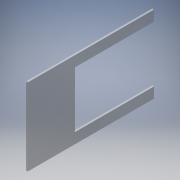
# Autodesk Inventor part: Inner side wall
Saved by Autodesk Inventor 2017 (Build 210142000, 142)
## iProperties
Created: 2017-09-30
Part Number: Inner side wall
Material: Glass
Document SubType Name: Modeling
Designer: Kenneth
Density: 2.18 g/cm^3
Appearance: Clear
Author: Kenneth
Autodesk Inventor part; units mm, degrees
ref_plane "YZ Plane" through (0, 0, 0) normal (1, 0, 0) x (0, 1, 0)
ref_plane "XZ Plane" through (0, 0, 0) normal (0, 1, 0) x (-1, 0, 0)
ref_plane "XY Plane" through (0, 0, 0) normal (0, 0, 1) x (1, 0, 0)
sketch "Sketch1" plane through (0, 0, 0) normal (1, 0, 0) x (0, 1, 0)
  line L0 (0, 0) -> (0, -457.2)
  line L1 (279.4, -457.2) -> (279.4, 0)
  line L2 (279.4, 0) -> (0, 0)
  line L3 (279.4, -457.2) -> (241.3, -457.2)
  line L4 (241.3, -457.2) -> (241.3, -171.0593)
  line L5 (241.3, -171.0593) -> (38.1, -171.0593)
  line L6 (38.1, -171.0593) -> (38.1, -457.2)
  line L7 (38.1, -457.2) -> (0, -457.2)
  dimension "d0" = 457.2
  dimension "d1" = 279.4
  dimension "d4" = 90
  dimension "d5" = 90
  dimension "dist1435" = 38.1
  dimension "d7" = 38.1
  constraints: 16 end point, 2 parallel, 1 horizontal, 1 perpendicular, 1 vertical
  measures "d0" distance of L1.start L1.end
  measures "d1" distance of L1.end L0.start
  measures "d4" angle of L6 L7
  measures "d5" angle of L5 L4
  measures "dist1435" distance of L1.start L3.end
  measures "d7" distance of L6.end L0.end
extrude "Extrusion1" add sketch "Sketch1" along normal blind 6.35
equation "\"d7\" = dist1435"
body "Solid1"
